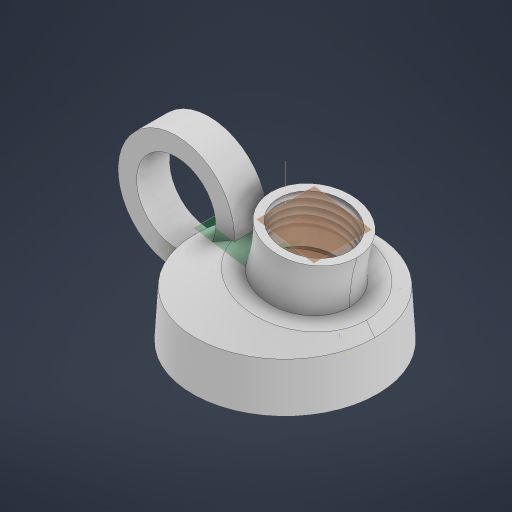
# Autodesk Inventor part: Część2
Saved by Autodesk Inventor 2023 (Build 270158000, 158)
## iProperties
Created: 2023-05-16
Part Number: Część2
Material: Ogólny
Document SubType Name: Modeling
Designer: Adam
Density: 1 g/cm^3
Appearance: Domyślna
Author: Adam
Autodesk Inventor part; units mm, degrees
ref_plane "YZ Plane" through (0, 0, 0) normal (1, 0, 0) x (0, 1, 0)
ref_plane "XZ Plane" through (0, 0, 0) normal (0, 1, 0) x (-1, 0, 0)
ref_plane "XY Plane" through (0, 0, 0) normal (0, 0, 1) x (1, 0, 0)
sketch "Szkic2" plane through (0, 0, 0) normal (0, 1, 0) x (-1, 0, 0)
  circle A0 centre (0, 0) radius 35
  circle A1 centre (0, 0) radius 30.5
  dimension "d2" = 70
  dimension "d3" = 61
  constraints: 2 centre point, 2 coincident
  measures "d2" diameter of A0
  measures "d3" diameter of A1
ref_plane "Płaszczyzna konstrukcyjna10" through (0, 18, 0) normal (0, 1, 0) x (-1, 0, 0)
sketch "Szkic4" plane through (0, 18, 0) normal (0, 1, 0) x (-1, 0, 0)
  circle A0 centre (0, 0) radius 30.5
  circle A1 centre (0, 0) radius 34
  dimension "d6" = 61
  dimension "d7" = 68
  constraints: 2 centre point, 2 coincident
  measures "d6" diameter of A0
  measures "d7" diameter of A1
loft "Wyciągnięcie złożone1" add profiles "Szkic2", "Szkic4" contours A0 | A1 / A0 | A1
sketch "Szkic5" plane through (0, 18, 0) normal (0, 1, 0) x (1, 0, 0)
  circle A0 centre (0, 0) radius 30.5
  dimension "d12" = 61
  constraints: 1 centre point, 1 coincident
  measures "d12" diameter of A0
extrude "Wyciągnięcie proste1" cut sketch "Szkic5" against normal through all
ref_plane "Płaszczyzna konstrukcyjna7" through (0, 18, 0) normal (0, 1, 0) x (-1, 0, 0)
sketch "Szkic6" plane through (0, 18, 0) normal (0, 1, 0) x (-1, 0, 0)
  point P0 (0, 0)
sketch "Szkic7" plane through (0, 0, 0) normal (0, 0, 1) x (1, 0, 0)
  point P0 (0, 0)
  point P1 (-34, 18)
ref_plane "Płaszczyzna konstrukcyjna4" through (0, 0, 10) normal (0, 0, 1) x (1, 0, 0)
sketch "Szkic8" plane through (0, 0, 10) normal (0, 0, 1) x (1, 0, 0)
  point P0 (0, 0)
ref_plane "Płaszczyzna konstrukcyjna8" through (0, 18, 0) normal (0, 1, 0) x (-1, 0, 0)
sketch "Szkic9" plane through (0, 18, 0) normal (0, 1, 0) x (-1, 0, 0)
  point P0 (0, 0)
ref_plane "Płaszczyzna konstrukcyjna9" through (0, 18, 0) normal (0, 1, 0) x (-1, 0, 0)
sketch "Szkic10" plane through (0, 18, 0) normal (0, 1, 0) x (-1, 0, 0)
  point P0 (0, 0)
ref_plane "Płaszczyzna konstrukcyjna5" through (0, 0, 10) normal (0, 0, 1) x (1, 0, 0)
sketch "Szkic11" plane through (0, 0, 10) normal (0, 0, 1) x (1, 0, 0)
  point P0 (0, 0)
ref_plane "Płaszczyzna konstrukcyjna18" through (0, 0, 10) normal (0, 0, 1) x (1, 0, 0)
sketch "Szkic12" plane through (0, 0, 10) normal (0, 0, 1) x (1, 0, 0)
  point P0 (0, 0)
  point P1 (-34, 18)
  point P2 (34, 18)
  point P3 (-12.7, 29)
  point P4 (30.69, 22)
ref_plane "Płaszczyzna konstrukcyjna11" through (-12.7, 29, 0) normal (-0.1592682, -0.9872354, 0) x (0.9872354, -0.1592682, 0)
sketch "Szkic13" plane through (-12.7, 29, 0) normal (-0.1592682, -0.9872354, 0) x (0.9872354, -0.1592682, 0)
  circle A0 centre (20.9386, -0.1965) radius 23
  line L0 (43.9505, 0) -> (44, 2)
  point P0 (17.1567, 0)
  dimension "d20" = 46
  constraints: 2 end point, 1 centre point, 1 tangent
  measures "d20" diameter of A0
loft "Wyciągnięcie złożone2" add profiles "Szkic13" section 1 edges at (34, 18, 0)
sketch "Szkic20" plane through (7.9713, 25.6652, -0.1965) normal (0.1592682, 0.9872354, 0) x (0.9872354, -0.1592682, 0)
  circle A0 centre (0, 0) radius 16.5
  point P0 (-3.7819, -0.1965)
  dimension "d37" = 33
  constraints: 1 centre point
  measures "d37" diameter of A0
ref_plane "Płaszczyzna konstrukcyjna17" through (9.4047, 34.5503, -0.1965) normal (0.1592682, 0.9872354, 0) x (0.9872354, -0.1592682, 0)
sketch "Szkic21" plane through (9.4047, 34.5503, -0.1965) normal (0.1592682, 0.9872354, 0) x (0.9872354, -0.1592682, 0)
  circle A0 centre (0, 0) radius 15.75
  point P0 (-3.7819, -0.1965)
  dimension "d39" = 31.5
  constraints: 1 centre point
  measures "d39" diameter of A0
ref_plane "Płaszczyzna konstrukcyjna15" through (10.8381, 43.4354, -0.1965) normal (0.1592682, 0.9872354, 0) x (0.9872354, -0.1592682, 0)
sketch "Szkic22" plane through (10.8381, 43.4354, -0.1965) normal (0.1592682, 0.9872354, 0) x (0.9872354, -0.1592682, 0)
  circle A0 centre (0, 0) radius 16.5
  point P0 (-3.7819, -0.1965)
  dimension "d41" = 33
  constraints: 1 centre point
  measures "d41" diameter of A0
loft "Wyciągnięcie złożone3" add profiles "Szkic20", "Szkic21", "Szkic22"
ref_plane "Płaszczyzna konstrukcyjna14" through (10.8381, 43.4354, -0.1965) normal (0.1592682, 0.9872354, 0) x (0.9872354, -0.1592682, 0)
sketch "Szkic23" plane through (10.8381, 43.4354, -0.1965) normal (0.1592682, 0.9872354, 0) x (0.9872354, -0.1592682, 0)
  point P0 (-3.7819, -0.1965)
  point P1 (0, 0)
hole "Otwór2" at (10.8381, 43.4354, -0.1965) direction (-0.1592682, -0.9872354, 0) diameter 27 end through all
thread "Gwint1" size "M27x3" class "6H" standard "ANSI Metric M Profile" length 13
sketch "Szkic24" plane through (0, 0, 0) normal (0, 0, 1) x (1, 0, 0)
  circle A0 centre (-35, 31) radius 22
  circle A1 centre (-35, 31) radius 15
  point P0 (0, 0)
  dimension "d57" = 44
  dimension "d58" = 30
  constraints: 2 centre point, 1 coincident
  measures "d57" diameter of A0
  measures "d58" diameter of A1
extrude "Wyciągnięcie proste3" add sketch "Szkic24" along normal mid plane 12.5
thread "Gwint2" size "M58x4" class "6H" standard "ANSI Metric M Profile" length 13
sketch "Szkic25" plane through (0, 0, 6.25) normal (0, 0, 1) x (1, 0, 0)
  point P0 (0, 0)
sketch "Szkic26" plane through (0, 0, 0) normal (0, 1, 0) x (-1, 0, 0)
  circle A0 centre (0, 0) radius 30.5
  constraints: 1 centre point, 1 coincident
extrude "Wyciągnięcie proste4" cut sketch "Szkic26" along normal blind 18
sketch "Szkic27" plane through (0, 18, 0) normal (0, -1, 0) x (1, 0, 0)
  circle A0 centre (0, 0) radius 20.5
  dimension "d65" = 41
  constraints: 1 centre point, 1 coincident
  measures "d65" diameter of A0
extrude "Wyciągnięcie proste5" cut sketch "Szkic27" against normal blind 6
sketch "Szkic28" plane through (0, 18, 0) normal (0, -1, 0) x (1, 0, 0)
  circle A0 centre (0, 0) radius 29
  circle A1 centre (0, 0) radius 21.5
  dimension "d68" = 58
  dimension "d70" = 43
  constraints: 2 centre point, 2 coincident
  measures "d68" diameter of A0
  measures "d70" diameter of A1
extrude "Wyciągnięcie proste6" cut sketch "Szkic28" against normal blind 2.5
sketch "Szkic29" plane through (-13.0855, 29.0622, 6.25) normal (0.1592682, 0.9872354, 0) x (0.9872354, -0.1592682, 0)
  point P0 (17.5472, 6.25)
sketch "Szkic30" plane through (0, 18, 0) normal (0, 1, 0) x (-1, 0, 0)
  point P0 (0, 0)
sketch "Szkic31" plane through (0, 20.5, 0) normal (0, -1, 0) x (1, 0, 0)
  circle A0 centre (0, 0) radius 27
  circle A1 centre (0, 0) radius 26.5
  dimension "d73" = 54
  dimension "d74" = 53
  constraints: 2 centre point, 2 coincident
  measures "d73" diameter of A0
  measures "d74" diameter of A1
extrude "Wyciągnięcie proste7" add sketch "Szkic31" along normal blind 2.5
sketch "Szkic32" plane through (0, 0, 0) normal (0, 0, 1) x (1, 0, 0)
  point P0 (0, 0)
sketch "Szkic33" plane through (0, 0, 0) normal (0, 0, 1) x (1, 0, 0)
  point P0 (0, 0)
sketch "Szkic34" plane through (0, 0, 0) normal (0, 0, 1) x (1, 0, 0)
  line L0 (-30.5, 18) -> (30.5, 18) projected
  line L1 (29, 20.5) -> (-29, 20.5) projected
  line L2 (-29, 18) -> (-29, 20.5)
  line L3 (-29, 20.5) -> (-21.4942, 20.5)
  line L4 (-21.5, 20.5) -> (-21.5, 18) projected
  line L5 (-21.5, 18) -> (-29, 18)
  point P0 (0, 0)
  constraints: 6 end point, 3 point on line, 1 perpendicular, 1 vertical
extrude "Żebro1" add sketch "Szkic34" along normal mid plane 1 rib yes fills toward (-25.25, 18.05) open curves L5 L2 L3
sketch "Szkic35" plane through (0, 18, 0) normal (0, -1, 0) x (1, 0, 0)
  circle A0 centre (0, 0) radius 20.5
  circle A1 centre (0, 0) radius 21.5
  constraints: 2 centre point, 2 coincident
extrude "Wyciągnięcie proste8" add sketch "Szkic35" along normal blind 2
ref_plane "Płaszczyzna konstrukcyjna16" through (7.6528, 23.6907, -0.1965) normal (0.1592682, 0.9872354, 0) x (0.9872354, -0.1592682, 0)
sketch "Szkic36" plane through (7.6528, 23.6907, -0.1965) normal (0.1592682, 0.9872354, 0) x (0.9872354, -0.1592682, 0)
  circle A0 centre (0, 0) radius 13.5 projected
  arc A1 (11.0483, 7.7578) -> (11.4118, -7.2125) centre (0, 0) ccw projected
  arc A2 (11.4118, 7.2125) -> (11.4118, -7.2125) centre (-5.0382, 0) ccw
  line L0 (11.4118, -7.2125) -> (11.4118, 7.2125) construction
  line L1 (11.4118, -7.2125) -> (25.8368, -7.2125) construction
  arc A3 (11.4118, 7.2125) -> (11.4118, -7.2125) centre (0, 0) ccw
  point P0 (-3.7819, -0.1965)
  point P1 (10.455, 8.5406)
  point P2 (10.455, -8.5406)
  dimension "d89" = 90
  constraints: 5 point on circle, 4 end point, 2 centre point, 1 concentric, 1 horizontal, 1 perpendicular
  measures "d89" angle of L1 L0
extrude "Wyciągnięcie proste9" cut sketch "Szkic36" against normal through all contours A0 A2
chamfer "Faza1" distance 3.35 angle 45 1 edges at (-15.5947, 24, -0.1965)
pattern_circular "Szyk kołowy2" count 44 over 360 about axis through (0, -10, 0) along (0, 1, 0) of "Żebro1"
